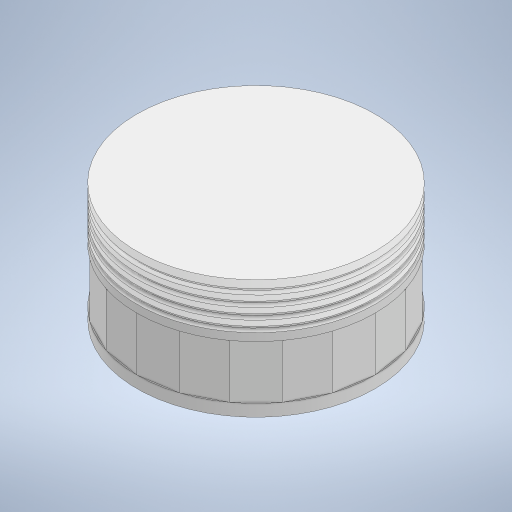
# Autodesk Inventor part: 援助上面
Saved by Autodesk Inventor 2024.2 (Build 282272000, 272)
## iProperties
Created: 2024-06-03
Part Number: 援助上面
Material: 一般
Document SubType Name: Modeling
Designer: sohil
Density: 1 g/cm^3
Appearance: 預設
Author: sohil
Autodesk Inventor part; units mm, degrees
ref_plane "YZ Plane" through (0, 0, 0) normal (1, 0, 0) x (0, 1, 0)
ref_plane "XZ Plane" through (0, 0, 0) normal (0, 1, 0) x (-1, 0, 0)
sketch "草圖1" plane through (0, 0, 0) normal (0, 1, 0) x (-1, 0, 0)
  circle A0 centre (0, 0) radius 15
  dimension "d0" = 30
  constraints: 1 centre point, 1 coincident
  measures "d0" diameter of A0
extrude "擠出1" add sketch "草圖1" along normal blind 1.5
sketch "草圖4" plane through (0, 1.5, 0) normal (0, 1, 0) x (1, 0, 0)
  circle A0 centre (0, 0) radius 15 projected
  line L0 (0, 15) -> (4.6353, 14.2658)
  line L1 (4.6353, 14.2658) -> (8.8168, 12.1353)
  line L2 (8.8168, 12.1353) -> (12.1353, 8.8168)
  line L3 (12.1353, 8.8168) -> (14.2658, 4.6353)
  line L4 (14.2658, 4.6353) -> (15, 0)
  line L5 (15, 0) -> (14.2658, -4.6353)
  line L6 (14.2658, -4.6353) -> (12.1353, -8.8168)
  line L7 (12.1353, -8.8168) -> (8.8168, -12.1353)
  line L8 (8.8168, -12.1353) -> (4.6353, -14.2658)
  line L9 (4.6353, -14.2658) -> (0, -15)
  line L10 (0, -15) -> (-4.6353, -14.2658)
  line L11 (-4.6353, -14.2658) -> (-8.8168, -12.1353)
  line L12 (-8.8168, -12.1353) -> (-12.1353, -8.8168)
  line L13 (-12.1353, -8.8168) -> (-14.2658, -4.6353)
  line L14 (-14.2658, -4.6353) -> (-15, 0)
  line L15 (-15, 0) -> (-14.2658, 4.6353)
  line L16 (-14.2658, 4.6353) -> (-12.1353, 8.8168)
  line L17 (-12.1353, 8.8168) -> (-8.8168, 12.1353)
  line L18 (-8.8168, 12.1353) -> (-4.6353, 14.2658)
  line L19 (-4.6353, 14.2658) -> (0, 15)
  constraints: 40 end point, 1 coincident, 1 vertical alignment, 42 other
extrude "擠出4" add sketch "草圖4" along normal blind 6.75 contours L5 L6 L7 L8 L9 L10 L11 L12 L13 L14 L15 L16 L17 L18 L19 L0 L1 L2 L3 L4
ref_plane "工作平面4" through (0, 1.5, 0) normal (-0.309, 0, 0.9511) x (0, 1, 0)
sketch "草圖6" plane through (0, 1.5, 0) normal (-0.309, 0, 0.9511) x (0, 1, 0)
  line L0 (6.75, 0) -> (6.75, 4.6353) projected
  line L1 (0, 15) -> (6.75, 15) projected
  line L2 (6.75, 0) -> (6.75, 15)
  line L3 (13.5, 15) -> (13.5, 0)
  line L4 (13.5, 0) -> (6.75, 0)
  line L5 (13.5, 15) -> (12.23, 15)
  line L6 (12.23, 15) -> (12.13, 15)
  line L7 (13.5, 15) -> (6.75, 15)
  line L8 (12.23, 15) -> (12.13, 15)
  line L9 (12.13, 15) -> (10.86, 15)
  line L10 (10.86, 15) -> (10.76, 15)
  line L11 (10.76, 15) -> (9.49, 15)
  line L12 (9.49, 15) -> (9.39, 15)
  line L13 (9.39, 15) -> (8.12, 15)
  line L14 (8.12, 15) -> (8.02, 15)
  line L15 (6.75, 14.2658) -> (6.75, 15) projected
  line L16 (8.02, 15) -> (6.75, 15)
  line L17 (12.13, 15) -> (12.23, 15)
  line L18 (12.23, 15) -> (12.23, 13)
  line L19 (12.23, 13) -> (12.13, 13)
  line L20 (12.13, 13) -> (12.13, 15)
  line L21 (10.76, 15) -> (10.86, 15)
  line L22 (10.86, 15) -> (10.86, 13)
  line L23 (10.86, 13) -> (10.76, 13)
  line L24 (10.76, 13) -> (10.76, 15)
  line L25 (9.49, 15) -> (9.39, 15)
  line L26 (9.39, 15) -> (9.39, 13)
  line L27 (9.39, 13) -> (9.49, 13)
  line L28 (9.49, 13) -> (9.49, 15)
  line L29 (8.12, 15) -> (8.02, 15)
  line L30 (8.02, 15) -> (8.02, 13)
  line L31 (8.02, 13) -> (8.12, 13)
  line L32 (8.12, 13) -> (8.12, 15)
  point P0 (-1.5, 0)
  point P1 (6.75, 4.6353)
  dimension "d17" = 1.27
  dimension "d24" = 0.1
  dimension "d25" = 1.27
  dimension "d26" = 0.1
  dimension "d27" = 1.27
  dimension "d28" = 0.1
  dimension "d29" = 1.27
  dimension "d30" = 0.1
  dimension "d31" = 1.27
  dimension "d32" = 2
  dimension "d33" = 2
  dimension "d34" = 2
  dimension "d35" = 2
  constraints: 60 end point, 9 parallel, 7 perpendicular, 6 point on line, 4 collinear, 1 horizontal
  measures "d17" distance of L3.start L5.end
  measures "d24" distance of L5.end L6.end
  measures "d25" distance of L6.end L9.end
  measures "d26" distance of L9.end L10.end
  measures "d27" distance of L10.end L11.end
  measures "d28" distance of L11.end L12.end
  measures "d29" distance of L12.end L13.end
  measures "d30" distance of L13.end L14.end
  measures "d31" distance of L14.end L1.end
  measures "d32" distance of L5.end L18.end
  measures "d33" distance of L9.end L22.end
  measures "d34" distance of L26.end L12.end
  measures "d35" distance of L30.end L14.end
revolve "迴轉1" add sketch "草圖6" angle 360 about axis through (0, 15, 0) along (0, -1, 0) contours L0 L2 L7 L30 L31 L32 L26 L27 L28 L24 L23 L22 L20 L19 L18 L5 L3 L4
fillet "圓角1" radius 0.3 8 edges at (14.2658, 13.73, 4.6353) (14.2658, 13.63, 4.6353) (14.2658, 12.36, 4.6353) (14.2658, 12.26, 4.6353) (14.2658, 10.99, 4.6353) (14.2658, 10.89, 4.6353) (14.2658, 9.62, 4.6353) (14.2658, 9.52, 4.6353)
